Autodesk Inventor part; units mm, degrees
(part 3 of 4)
  line L1517 (59.25, 16.75) -> (45.25, 30.75) construction
  line L1518 (78.25, 16.75) -> (78.25, 30.75)
  line L1519 (64.25, 30.75) -> (64.25, 16.75)
  line L1520 (78.25, 30.75) -> (64.25, 30.75)
  line L1521 (64.25, 16.75) -> (78.25, 16.75)
  line L1522 (64.25, 16.75) -> (78.25, 30.75) construction
  line L1523 (78.25, 16.75) -> (64.25, 30.75) construction
  line L1524 (97.25, 16.75) -> (97.25, 30.75)
  line L1525 (83.25, 30.75) -> (83.25, 16.75)
  line L1526 (97.25, 30.75) -> (83.25, 30.75)
  line L1527 (83.25, 16.75) -> (97.25, 16.75)
  line L1528 (83.25, 16.75) -> (97.25, 30.75) construction
  line L1529 (97.25, 16.75) -> (83.25, 30.75) construction
  line L1530 (116.25, 16.75) -> (116.25, 30.75)
  line L1531 (102.25, 30.75) -> (102.25, 16.75)
  line L1532 (116.25, 30.75) -> (102.25, 30.75)
  line L1533 (102.25, 16.75) -> (116.25, 16.75)
  line L1534 (102.25, 16.75) -> (116.25, 30.75) construction
  line L1535 (116.25, 16.75) -> (102.25, 30.75) construction
  line L1536 (135.25, 16.75) -> (135.25, 30.75)
  line L1537 (121.25, 30.75) -> (121.25, 16.75)
  line L1538 (135.25, 30.75) -> (121.25, 30.75)
  line L1539 (121.25, 16.75) -> (135.25, 16.75)
  line L1540 (121.25, 16.75) -> (135.25, 30.75) construction
  line L1541 (135.25, 16.75) -> (121.25, 30.75) construction
  line L1542 (154.25, 16.75) -> (154.25, 30.75)
  line L1543 (140.25, 30.75) -> (140.25, 16.75)
  line L1544 (154.25, 30.75) -> (140.25, 30.75)
  line L1545 (140.25, 16.75) -> (154.25, 16.75)
  line L1546 (140.25, 16.75) -> (154.25, 30.75) construction
  line L1547 (154.25, 16.75) -> (140.25, 30.75) construction
  line L1548 (173.25, 16.75) -> (173.25, 30.75)
  line L1549 (159.25, 30.75) -> (159.25, 16.75)
  line L1550 (173.25, 30.75) -> (159.25, 30.75)
  line L1551 (159.25, 16.75) -> (173.25, 16.75)
  line L1552 (159.25, 16.75) -> (173.25, 30.75) construction
  line L1553 (173.25, 16.75) -> (159.25, 30.75) construction
  line L1554 (-64, -2.25) -> (-50, -2.25)
  line L1555 (-50, -2.25) -> (-50, 11.75)
  line L1556 (-50, 11.75) -> (-64, 11.75)
  line L1557 (-64, 11.75) -> (-64, -2.25)
  line L1558 (-64, -2.25) -> (-50, 11.75) construction
  line L1559 (-50, -2.25) -> (-64, 11.75) construction
  line L1560 (-61.625, -21.25) -> (-47.625, -21.25)
  line L1561 (-47.625, -21.25) -> (-47.625, -7.25)
  line L1562 (-47.625, -7.25) -> (-61.625, -7.25)
  line L1563 (-61.625, -7.25) -> (-61.625, -21.25)
  line L1564 (-61.625, -21.25) -> (-47.625, -7.25) construction
  line L1565 (-47.625, -21.25) -> (-61.625, -7.25) construction
  line L1566 (-56.875, -40.25) -> (-42.875, -40.25)
  line L1567 (-42.875, -40.25) -> (-42.875, -26.25)
  line L1568 (-42.875, -26.25) -> (-56.875, -26.25)
  line L1569 (-56.875, -26.25) -> (-56.875, -40.25)
  line L1570 (-56.875, -40.25) -> (-42.875, -26.25) construction
  line L1571 (-42.875, -40.25) -> (-56.875, -26.25) construction
  line L1572 (-66.375, -59.25) -> (-52.375, -59.25)
  line L1573 (-52.375, -59.25) -> (-52.375, -45.25)
  line L1574 (-52.375, -45.25) -> (-66.375, -45.25)
  line L1575 (-66.375, -45.25) -> (-66.375, -59.25)
  line L1576 (-66.375, -59.25) -> (-52.375, -45.25) construction
  line L1577 (-52.375, -59.25) -> (-66.375, -45.25) construction
  line L1578 (-42.625, -59.25) -> (-28.625, -59.25)
  line L1579 (-28.625, -59.25) -> (-28.625, -45.25)
  line L1580 (-28.625, -45.25) -> (-42.625, -45.25)
  line L1581 (-42.625, -45.25) -> (-42.625, -59.25)
  line L1582 (-42.625, -59.25) -> (-28.625, -45.25) construction
  line L1583 (-28.625, -59.25) -> (-42.625, -45.25) construction
  line L1584 (-18.875, -59.25) -> (-4.875, -59.25)
  line L1585 (-4.875, -59.25) -> (-4.875, -45.25)
  line L1586 (-4.875, -45.25) -> (-18.875, -45.25)
  line L1587 (-18.875, -45.25) -> (-18.875, -59.25)
  line L1588 (-18.875, -59.25) -> (-4.875, -45.25) construction
  line L1589 (-4.875, -59.25) -> (-18.875, -45.25) construction
  line L1590 (64.25, -59.25) -> (78.25, -59.25)
  line L1591 (78.25, -59.25) -> (78.25, -45.25)
  line L1592 (78.25, -45.25) -> (64.25, -45.25)
  line L1593 (64.25, -45.25) -> (64.25, -59.25)
  line L1594 (64.25, -59.25) -> (78.25, -45.25) construction
  line L1595 (78.25, -59.25) -> (64.25, -45.25) construction
  line L1596 (147.375, -59.25) -> (161.375, -59.25)
  line L1597 (161.375, -59.25) -> (161.375, -45.25)
  line L1598 (161.375, -45.25) -> (147.375, -45.25)
  line L1599 (147.375, -45.25) -> (147.375, -59.25)
  line L1600 (147.375, -59.25) -> (161.375, -45.25) construction
  line L1601 (161.375, -59.25) -> (147.375, -45.25) construction
  line L1602 (171.125, -59.25) -> (185.125, -59.25)
  line L1603 (185.125, -59.25) -> (185.125, -45.25)
  line L1604 (185.125, -45.25) -> (171.125, -45.25)
  line L1605 (171.125, -45.25) -> (171.125, -59.25)
  line L1606 (171.125, -59.25) -> (185.125, -45.25) construction
  line L1607 (185.125, -59.25) -> (171.125, -45.25) construction
  line L1608 (194.875, -59.25) -> (208.875, -59.25)
  line L1609 (208.875, -59.25) -> (208.875, -45.25)
  line L1610 (208.875, -45.25) -> (194.875, -45.25)
  line L1611 (194.875, -45.25) -> (194.875, -59.25)
  line L1612 (194.875, -59.25) -> (208.875, -45.25) construction
  line L1613 (208.875, -59.25) -> (194.875, -45.25) construction
  line L1614 (180.625, -40.25) -> (194.625, -40.25)
  line L1615 (194.625, -40.25) -> (194.625, -26.25)
  line L1616 (194.625, -26.25) -> (180.625, -26.25)
  line L1617 (180.625, -26.25) -> (180.625, -40.25)
  line L1618 (180.625, -40.25) -> (194.625, -26.25) construction
  line L1619 (194.625, -40.25) -> (180.625, -26.25) construction
  line L1620 (185.375, -21.25) -> (199.375, -21.25)
  line L1621 (199.375, -21.25) -> (199.375, -7.25)
  line L1622 (199.375, -7.25) -> (185.375, -7.25)
  line L1623 (185.375, -7.25) -> (185.375, -21.25)
  line L1624 (185.375, -21.25) -> (199.375, -7.25) construction
  line L1625 (199.375, -21.25) -> (185.375, -7.25) construction
  line L1626 (192.5, -2.25) -> (206.5, -2.25)
  line L1627 (206.5, -2.25) -> (206.5, 11.75)
  line L1628 (206.5, 11.75) -> (192.5, 11.75)
  line L1629 (192.5, 11.75) -> (192.5, -2.25)
  line L1630 (192.5, -2.25) -> (206.5, 11.75) construction
  line L1631 (206.5, -2.25) -> (192.5, 11.75) construction
  line L1632 (187.75, 16.75) -> (201.75, 16.75)
  line L1633 (201.75, 16.75) -> (201.75, 30.75)
  line L1634 (201.75, 30.75) -> (187.75, 30.75)
  line L1635 (187.75, 30.75) -> (187.75, 16.75)
  line L1636 (187.75, 16.75) -> (201.75, 30.75) construction
  line L1637 (201.75, 16.75) -> (187.75, 30.75) construction
  line L1638 (-40.25, -2.25) -> (-26.25, -2.25)
  line L1639 (-26.25, -2.25) -> (-26.25, 11.75)
  line L1640 (-26.25, 11.75) -> (-40.25, 11.75)
  line L1641 (-40.25, 11.75) -> (-40.25, -2.25)
  line L1642 (-40.25, -2.25) -> (-26.25, 11.75) construction
  line L1643 (-26.25, -2.25) -> (-40.25, 11.75) construction
  line L1644 (-35.5, -21.25) -> (-21.5, -21.25)
  line L1645 (-21.5, -21.25) -> (-21.5, -7.25)
  line L1646 (-21.5, -7.25) -> (-35.5, -7.25)
  line L1647 (-35.5, -7.25) -> (-35.5, -21.25)
  line L1648 (-35.5, -21.25) -> (-21.5, -7.25) construction
  line L1649 (-21.5, -21.25) -> (-35.5, -7.25) construction
  line L1650 (-26, -40.25) -> (-12, -40.25)
  line L1651 (-12, -40.25) -> (-12, -26.25)
  line L1652 (-12, -26.25) -> (-26, -26.25)
  line L1653 (-26, -26.25) -> (-26, -40.25)
  line L1654 (-26, -40.25) -> (-12, -26.25) construction
  line L1655 (-12, -40.25) -> (-26, -26.25) construction
  line L1656 (-21.25, -2.25) -> (-7.25, -2.25)
  line L1657 (-21.25, 11.75) -> (-21.25, -2.25)
  line L1658 (-7.25, -2.25) -> (-7.25, 11.75)
  line L1659 (-7.25, 11.75) -> (-21.25, 11.75)
  line L1660 (-21.25, -2.25) -> (-7.25, 11.75) construction
  line L1661 (-7.25, -2.25) -> (-21.25, 11.75) construction
  line L1662 (-2.25, -2.25) -> (11.75, -2.25)
  line L1663 (-2.25, 11.75) -> (-2.25, -2.25)
  line L1664 (11.75, -2.25) -> (11.75, 11.75)
  line L1665 (11.75, 11.75) -> (-2.25, 11.75)
  line L1666 (-2.25, -2.25) -> (11.75, 11.75) construction
  line L1667 (11.75, -2.25) -> (-2.25, 11.75) construction
  line L1668 (16.75, -2.25) -> (30.75, -2.25)
  line L1669 (16.75, 11.75) -> (16.75, -2.25)
  line L1670 (30.75, -2.25) -> (30.75, 11.75)
  line L1671 (30.75, 11.75) -> (16.75, 11.75)
  line L1672 (16.75, -2.25) -> (30.75, 11.75) construction
  line L1673 (30.75, -2.25) -> (16.75, 11.75) construction
  line L1674 (35.75, -2.25) -> (49.75, -2.25)
  line L1675 (35.75, 11.75) -> (35.75, -2.25)
  line L1676 (49.75, -2.25) -> (49.75, 11.75)
  line L1677 (49.75, 11.75) -> (35.75, 11.75)
  line L1678 (35.75, -2.25) -> (49.75, 11.75) construction
  line L1679 (49.75, -2.25) -> (35.75, 11.75) construction
  line L1680 (54.75, -2.25) -> (68.75, -2.25)
  line L1681 (54.75, 11.75) -> (54.75, -2.25)
  line L1682 (68.75, -2.25) -> (68.75, 11.75)
  line L1683 (68.75, 11.75) -> (54.75, 11.75)
  line L1684 (54.75, -2.25) -> (68.75, 11.75) construction
  line L1685 (68.75, -2.25) -> (54.75, 11.75) construction
  line L1686 (73.75, -2.25) -> (87.75, -2.25)
  line L1687 (73.75, 11.75) -> (73.75, -2.25)
  line L1688 (87.75, -2.25) -> (87.75, 11.75)
  line L1689 (87.75, 11.75) -> (73.75, 11.75)
  line L1690 (73.75, -2.25) -> (87.75, 11.75) construction
  line L1691 (87.75, -2.25) -> (73.75, 11.75) construction
  line L1692 (92.75, -2.25) -> (106.75, -2.25)
  line L1693 (92.75, 11.75) -> (92.75, -2.25)
  line L1694 (106.75, -2.25) -> (106.75, 11.75)
  line L1695 (106.75, 11.75) -> (92.75, 11.75)
  line L1696 (92.75, -2.25) -> (106.75, 11.75) construction
  line L1697 (106.75, -2.25) -> (92.75, 11.75) construction
  line L1698 (111.75, -2.25) -> (125.75, -2.25)
  line L1699 (111.75, 11.75) -> (111.75, -2.25)
  line L1700 (125.75, -2.25) -> (125.75, 11.75)
  line L1701 (125.75, 11.75) -> (111.75, 11.75)
  line L1702 (111.75, -2.25) -> (125.75, 11.75) construction
  line L1703 (125.75, -2.25) -> (111.75, 11.75) construction
  line L1704 (130.75, -2.25) -> (144.75, -2.25)
  line L1705 (130.75, 11.75) -> (130.75, -2.25)
  line L1706 (144.75, -2.25) -> (144.75, 11.75)
  line L1707 (144.75, 11.75) -> (130.75, 11.75)
  line L1708 (130.75, -2.25) -> (144.75, 11.75) construction
  line L1709 (144.75, -2.25) -> (130.75, 11.75) construction
  line L1710 (149.75, -2.25) -> (163.75, -2.25)
  line L1711 (149.75, 11.75) -> (149.75, -2.25)
  line L1712 (163.75, -2.25) -> (163.75, 11.75)
  line L1713 (163.75, 11.75) -> (149.75, 11.75)
  line L1714 (149.75, -2.25) -> (163.75, 11.75) construction
  line L1715 (163.75, -2.25) -> (149.75, 11.75) construction
  line L1716 (168.75, -2.25) -> (182.75, -2.25)
  line L1717 (168.75, 11.75) -> (168.75, -2.25)
  line L1718 (182.75, -2.25) -> (182.75, 11.75)
  line L1719 (182.75, 11.75) -> (168.75, 11.75)
  line L1720 (168.75, -2.25) -> (182.75, 11.75) construction
  line L1721 (182.75, -2.25) -> (168.75, 11.75) construction
  line L1722 (-16.5, -21.25) -> (-2.5, -21.25)
  line L1723 (-16.5, -7.25) -> (-16.5, -21.25)
  line L1724 (-2.5, -7.25) -> (-16.5, -7.25)
  line L1725 (-2.5, -21.25) -> (-2.5, -7.25)
  line L1726 (-16.5, -21.25) -> (-2.5, -7.25) construction
  line L1727 (-2.5, -21.25) -> (-16.5, -7.25) construction
  line L1728 (2.5, -21.25) -> (16.5, -21.25)
  line L1729 (2.5, -7.25) -> (2.5, -21.25)
  line L1730 (16.5, -7.25) -> (2.5, -7.25)
  line L1731 (16.5, -21.25) -> (16.5, -7.25)
  line L1732 (2.5, -21.25) -> (16.5, -7.25) construction
  line L1733 (16.5, -21.25) -> (2.5, -7.25) construction
  line L1734 (21.5, -21.25) -> (35.5, -21.25)
  line L1735 (21.5, -7.25) -> (21.5, -21.25)
  line L1736 (35.5, -7.25) -> (21.5, -7.25)
  line L1737 (35.5, -21.25) -> (35.5, -7.25)
  line L1738 (21.5, -21.25) -> (35.5, -7.25) construction
  line L1739 (35.5, -21.25) -> (21.5, -7.25) construction
  line L1740 (40.5, -21.25) -> (54.5, -21.25)
  line L1741 (40.5, -7.25) -> (40.5, -21.25)
  line L1742 (54.5, -7.25) -> (40.5, -7.25)
  line L1743 (54.5, -21.25) -> (54.5, -7.25)
  line L1744 (40.5, -21.25) -> (54.5, -7.25) construction
  line L1745 (54.5, -21.25) -> (40.5, -7.25) construction
  line L1746 (59.5, -21.25) -> (73.5, -21.25)
  line L1747 (59.5, -7.25) -> (59.5, -21.25)
  line L1748 (73.5, -7.25) -> (59.5, -7.25)
  line L1749 (73.5, -21.25) -> (73.5, -7.25)
  line L1750 (59.5, -21.25) -> (73.5, -7.25) construction
  line L1751 (73.5, -21.25) -> (59.5, -7.25) construction
  line L1752 (78.5, -21.25) -> (92.5, -21.25)
  line L1753 (78.5, -7.25) -> (78.5, -21.25)
  line L1754 (92.5, -7.25) -> (78.5, -7.25)
  line L1755 (92.5, -21.25) -> (92.5, -7.25)
  line L1756 (78.5, -21.25) -> (92.5, -7.25) construction
  line L1757 (92.5, -21.25) -> (78.5, -7.25) construction
  line L1758 (97.5, -21.25) -> (111.5, -21.25)
  line L1759 (97.5, -7.25) -> (97.5, -21.25)
  line L1760 (111.5, -7.25) -> (97.5, -7.25)
  line L1761 (111.5, -21.25) -> (111.5, -7.25)
  line L1762 (97.5, -21.25) -> (111.5, -7.25) construction
  line L1763 (111.5, -21.25) -> (97.5, -7.25) construction
  line L1764 (116.5, -21.25) -> (130.5, -21.25)
  line L1765 (116.5, -7.25) -> (116.5, -21.25)
  line L1766 (130.5, -7.25) -> (116.5, -7.25)
  line L1767 (130.5, -21.25) -> (130.5, -7.25)
  line L1768 (116.5, -21.25) -> (130.5, -7.25) construction
  line L1769 (130.5, -21.25) -> (116.5, -7.25) construction
  line L1770 (135.5, -21.25) -> (149.5, -21.25)
  line L1771 (135.5, -7.25) -> (135.5, -21.25)
  line L1772 (149.5, -7.25) -> (135.5, -7.25)
  line L1773 (149.5, -21.25) -> (149.5, -7.25)
  line L1774 (135.5, -21.25) -> (149.5, -7.25) construction
  line L1775 (149.5, -21.25) -> (135.5, -7.25) construction
  line L1776 (154.5, -21.25) -> (168.5, -21.25)
  line L1777 (154.5, -7.25) -> (154.5, -21.25)
  line L1778 (168.5, -7.25) -> (154.5, -7.25)
  line L1779 (168.5, -21.25) -> (168.5, -7.25)
  line L1780 (154.5, -21.25) -> (168.5, -7.25) construction
  line L1781 (168.5, -21.25) -> (154.5, -7.25) construction
  line L1782 (-7, -40.25) -> (7, -40.25)
  line L1783 (-7, -26.25) -> (-7, -40.25)
  line L1784 (7, -26.25) -> (-7, -26.25)
  line L1785 (7, -40.25) -> (7, -26.25)
  line L1786 (-7, -40.25) -> (7, -26.25) construction
  line L1787 (7, -40.25) -> (-7, -26.25) construction
  line L1788 (12, -40.25) -> (26, -40.25)
  line L1789 (12, -26.25) -> (12, -40.25)
  line L1790 (26, -26.25) -> (12, -26.25)
  line L1791 (26, -40.25) -> (26, -26.25)
  line L1792 (12, -40.25) -> (26, -26.25) construction
  line L1793 (26, -40.25) -> (12, -26.25) construction
  line L1794 (31, -40.25) -> (45, -40.25)
  line L1795 (31, -26.25) -> (31, -40.25)
  line L1796 (45, -26.25) -> (31, -26.25)
  line L1797 (45, -40.25) -> (45, -26.25)
  line L1798 (31, -40.25) -> (45, -26.25) construction
  line L1799 (45, -40.25) -> (31, -26.25) construction
  line L1800 (50, -40.25) -> (64, -40.25)
  line L1801 (50, -26.25) -> (50, -40.25)
  line L1802 (64, -26.25) -> (50, -26.25)
  line L1803 (64, -40.25) -> (64, -26.25)
  line L1804 (50, -40.25) -> (64, -26.25) construction
  line L1805 (64, -40.25) -> (50, -26.25) construction
  line L1806 (69, -40.25) -> (83, -40.25)
  line L1807 (69, -26.25) -> (69, -40.25)
  line L1808 (83, -26.25) -> (69, -26.25)
  line L1809 (83, -40.25) -> (83, -26.25)
  line L1810 (69, -40.25) -> (83, -26.25) construction
  line L1811 (83, -40.25) -> (69, -26.25) construction
  line L1812 (88, -40.25) -> (102, -40.25)
  line L1813 (88, -26.25) -> (88, -40.25)
  line L1814 (102, -26.25) -> (88, -26.25)
  line L1815 (102, -40.25) -> (102, -26.25)
  line L1816 (88, -40.25) -> (102, -26.25) construction
  line L1817 (102, -40.25) -> (88, -26.25) construction
  line L1818 (107, -40.25) -> (121, -40.25)
  line L1819 (107, -26.25) -> (107, -40.25)
  line L1820 (121, -26.25) -> (107, -26.25)
  line L1821 (121, -40.25) -> (121, -26.25)
  line L1822 (107, -40.25) -> (121, -26.25) construction
  line L1823 (121, -40.25) -> (107, -26.25) construction
  line L1824 (126, -40.25) -> (140, -40.25)
  line L1825 (126, -26.25) -> (126, -40.25)
  line L1826 (140, -26.25) -> (126, -26.25)
  line L1827 (140, -40.25) -> (140, -26.25)
  line L1828 (126, -40.25) -> (140, -26.25) construction
  line L1829 (140, -40.25) -> (126, -26.25) construction
  line L1830 (145, -40.25) -> (159, -40.25)
  line L1831 (145, -26.25) -> (145, -40.25)
  line L1832 (159, -26.25) -> (145, -26.25)
  line L1833 (159, -40.25) -> (159, -26.25)
  line L1834 (145, -40.25) -> (159, -26.25) construction
  line L1835 (159, -40.25) -> (145, -26.25) construction
  point P0 (107.46, 92.5006)
  point P1 (-61.75, 52.25)
  point P2 (-23.75, 52.25)
  point P3 (-4.75, 52.25)
  point P4 (14.25, 52.25)
  point P5 (33.25, 52.25)
  point P6 (61.75, 52.25)
  point P7 (147.25, 52.25)
  point P8 (-204.25, 23.75)
  point P9 (-147.25, 23.75)
  point P10 (-147.25, -4.75)
  point P11 (-147.25, -42.75)
  point P12 (-123.5, -52.25)
  point P13 (-104.5, -52.25)
  point P14 (-85.5, -52.25)
  point P15 (-104.5, -33.25)
  point P16 (-123.5, 23.75)
  point P17 (-61.75, 23.75)
  point P18 (-57, 4.75)
  point P19 (-54.625, -14.25)
  point P20 (-49.875, -33.25)
  point P21 (-59.375, -52.25)
  point P22 (-35.625, -52.25)
  point P23 (-11.875, -52.25)
  point P24 (71.25, -52.25)
  point P25 (154.375, -52.25)
  point P26 (178.125, -52.25)
  point P27 (201.875, -52.25)
  point P28 (187.625, -33.25)
  point P29 (192.375, -14.25)
  point P30 (199.5, 4.75)
  point P31 (194.75, 23.75)
  point P32 (-33.25, 4.75)
  point P33 (-28.5, -14.25)
  point P34 (-19, -33.25)
  dimension "d0" = 0.7
  dimension "d1" = 0.7
  dimension "d2" = 14
  dimension "d3" = 14
  dimension "d4" = 14
  dimension "d5" = 14
  dimension "d6" = 14
  dimension "d7" = 14
  dimension "d8" = 14
  dimension "d9" = 14
  dimension "d10" = 14
  dimension "d11" = 14
  dimension "d12" = 14
  dimension "d13" = 14
  dimension "d16" = 19
  dimension "d21" = 14
  dimension "d22" = 14
  dimension "d25" = 19
  dimension "d30" = 14
  dimension "d31" = 14
  dimension "d34" = 19
  dimension "d37" = 19
  dimension "d40" = 14
  dimension "d41" = 14
  dimension "d42" = 14
  dimension "d43" = 14
  dimension "d44" = 14
  dimension "d45" = 14
  dimension "d46" = 14
  dimension "d47" = 14
  dimension "d48" = 14
  dimension "d49" = 14
  dimension "d50" = 14
  dimension "d51" = 14
  dimension "d52" = 14
  dimension "d53" = 14
  dimension "d54" = 14
  dimension "d55" = 14
  dimension "d58" = 19
  dimension "d61" = 19
  dimension "d64" = 14
  dimension "d65" = 14
  dimension "d68" = 19
  dimension "d73" = 14
  dimension "d74" = 14
  dimension "d75" = 14
  dimension "d76" = 14
  dimension "d77" = 14
  dimension "d78" = 14
  dimension "d79" = 14
  dimension "d80" = 14
  dimension "d81" = 14
  dimension "d82" = 14
  dimension "d83" = 14
  dimension "d84" = 14
  dimension "d85" = 14
  dimension "d86" = 14
  dimension "d87" = 14
  dimension "d88" = 14
  dimension "d89" = 14
  dimension "d90" = 14
  dimension "d91" = 14
  dimension "d92" = 14
  dimension "d93" = 14
  constraints: 1226 end point, 68 midpoint, 68 parallel, 43 horizontal, 38 perpendicular, 10 collinear, 5 point on line, 3 vertical, 660 other
  measures "d0" distance of L4.start L12.end
  measures "d1" distance of L4.end L15.end
  measures "d2" distance of L1232.end L1231.end
  measures "d3" distance of L1231.end L1230.end
  measures "d4" distance of L1238.end L1237.end
  measures "d5" distance of L1237.end L1236.end
  measures "d6" distance of L1244.end L1243.end
  measures "d7" distance of L1243.end L1242.end
  measures "d8" distance of L1250.end L1249.end
  measures "d9" distance of L1249.end L1248.end
  measures "d10" distance of L1256.end L1255.end
  measures "d11" distance of L1255.end L1254.end
  measures "d12" distance of L1262.end L1261.end
  measures "d13" distance of L1261.end L1260.end
  measures "d16" distance of L1260.start L1266.start
  measures "d21" distance of L1286.end L1285.end
  measures "d22" distance of L1285.end L1284.end
  measures "d25" distance of L1284.end L1290.start
  measures "d30" distance of L1310.end L1309.end
  measures "d31" distance of L1309.end L1308.end
  measures "d34" distance of L1309.end L1314.start
  measures "d37" distance of L1309.end L1326.start
  measures "d40" distance of L1400.end L1399.end
  measures "d41" distance of L1399.end L1398.end
  measures "d42" distance of L1406.end L1405.end
  measures "d43" distance of L1405.end L1404.end
  measures "d44" distance of L1412.end L1411.end
  measures "d45" distance of L1411.end L1410.end
  measures "d46" distance of L1418.end L1417.end
  measures "d47" distance of L1417.end L1416.end
  measures "d48" distance of L1424.end L1423.end
  measures "d49" distance of L1423.end L1422.end
  measures "d50" distance of L1430.end L1429.end
  measures "d51" distance of L1429.end L1428.end
  measures "d52" distance of L1435.end L1436.end
  measures "d53" distance of L1434.end L1435.end
  measures "d54" distance of L1442.end L1441.end
  measures "d55" distance of L1441.end L1440.end
  measures "d58" distance of L1442.end L1446.end
  measures "d61" distance of L1442.end L1458.end
  measures "d64" distance of L1478.end L1477.end
  measures "d65" distance of L1477.end L1476.end
  measures "d68" distance of L1476.end L1482.start
  measures "d73" distance of L1556.end L1555.end
  measures "d74" distance of L1555.end L1554.end
  measures "d75" distance of L1562.end L1561.end
  measures "d76" distance of L1561.end L1560.end
  measures "d77" distance of L1568.end L1567.end
  measures "d78" distance of L1567.end L1566.end
  measures "d79" distance of L1574.end L1573.end
  measures "d80" distance of L1573.end L1572.end
  measures "d81" distance of L1580.end L1579.end
  measures "d82" distance of L1579.end L1578.end
  measures "d83" distance of L1586.end L1585.end
  measures "d84" distance of L1585.end L1584.end
  measures "d85" distance of L1592.end L1591.end
  measures "d86" distance of L1591.end L1590.end
  measures "d87" distance of L1598.end L1597.end
  measures "d88" distance of L1597.end L1596.end
  measures "d89" distance of L1604.end L1603.end
  measures "d90" distance of L1603.end L1602.end
  measures "d91" distance of L1610.end L1609.end
  measures "d92" distance of L1609.end L1608.end
  measures "d93" distance of L1616.end L1615.end
extrude "Extrusion1" add sketch "Sketch1" against normal blind 1.5 contours A3 L3 A2 L2 A1 L1 A0 L0 | A4 | A5 | A6 | A7 | A8 | A9 | A10 | A11 | A12 | A13 | A14 | A15 | A16 | A17 | A18 | A19 | A20 | A21 | A22 | A23 | A24 | A25 | A26 | A27
sketch "Sketch2" plane through (-107.46, -92.5006, 10.9251) normal (0, 0, 1) x (1, 0, 0)
  arc A0 (-216.125, 61.75) -> (-220.875, 57) centre (-216.125, 57) ccw construction
  line L0 (-216.125, -61.75) -> (216.125, -61.75) construction
  line L1 (-220.875, 57) -> (-220.875, -57) construction
  arc A1 (220.875, 57) -> (216.125, 61.75) centre (216.125, 57) ccw construction
  line L2 (216.125, 61.75) -> (-216.125, 61.75) construction
  line L3 (-213.77, 61.75) -> (-213.77, -61.75) construction
  line L4 (-211.25, 30.75) -> (-197.25, 30.75) construction
  line L5 (-213.77, 35.75) -> (-212.3378, 39.685)
  line L6 (-205.2313, 59.21) -> (-202.7313, 59.21)
  line L7 (-213.77, 35.75) -> (-211.27, 35.75)
  line L8 (-210.231, 59.21) -> (-185.2654, 59.21) construction
  line L9 (-133.77, 35.75) -> (-108.8044, 35.75) construction
  line L10 (-128.77, 35.75) -> (-133.77, 35.75)
  line L11 (-123.77, 35.75) -> (-98.8044, 35.75) construction
  line L12 (-123.77, 35.75) -> (-118.77, 35.75)
  line L13 (-113.77, 35.75) -> (-88.8044, 35.75) construction
  line L14 (-108.77, 35.75) -> (-113.77, 35.75)
  line L15 (-103.77, 35.75) -> (-78.8044, 35.75) construction
  line L16 (-98.77, 35.75) -> (-103.77, 35.75)
  line L17 (-88.77, 35.75) -> (-93.77, 35.75)
  line L18 (-78.77, 35.75) -> (-83.77, 35.75)
  line L19 (-77.34, 41.535) -> (-77.34, 39.685) construction
  line L20 (-212.3378, 39.685) -> (-209.8378, 39.685)
  line L21 (-211.6644, 41.535) -> (-209.1644, 41.535)
  line L22 (-132.3378, 39.685) -> (-77.34, 39.685)
  line L23 (-77.34, 39.685) -> (-78.7722, 35.75)
  line L24 (-128.77, 35.75) -> (-123.77, 35.75)
  line L25 (-118.77, 35.75) -> (-113.77, 35.75)
  line L26 (-108.77, 35.75) -> (-103.77, 35.75)
  line L27 (-98.77, 35.75) -> (-93.77, 35.75)
  line L28 (-88.77, 35.75) -> (-83.77, 35.75)
  line L29 (-132.3378, 39.685) -> (-133.77, 35.75)
  line L30 (-211.6644, 41.535) -> (-205.2313, 59.21)
  line L31 (-129.54, 41.535) -> (-129.54, 59.315) construction
  line L32 (-129.54, 59.0513) -> (-131.39, 59.0513) construction
  line L33 (-129.54, 59.0513) -> (-127.69, 59.0513) construction
  line L34 (-131.39, 61.75) -> (-131.39, 56.0264) construction
  line L35 (-130.2313, 59.21) -> (220.875, 59.21) construction
  line L36 (-131.39, 56.0264) -> (-131.39, 39.685) construction
  line L37 (-211.27, 35.75) -> (-209.8378, 39.685) construction
  line L38 (-209.1644, 41.535) -> (-202.7313, 59.21) construction
  line L39 (-211.27, 35.75) -> (-209.8378, 39.685)
  line L40 (-209.1644, 41.535) -> (-202.7313, 59.21)
  line L41 (-213.77, 59.21) -> (-131.39, 59.21) construction
  line L42 (-200.2313, 59.21) -> (-197.7313, 59.21)
  line L43 (-204.1644, 41.535) -> (-197.7313, 59.21) construction
  line L44 (-204.1644, 41.535) -> (-197.7313, 59.21)
  line L45 (-206.6644, 41.535) -> (-200.2313, 59.21)
  line L46 (-206.6644, 41.535) -> (-204.1644, 41.535)
  line L47 (-207.3378, 39.685) -> (-204.8378, 39.685)
  line L48 (-206.27, 35.75) -> (-204.8378, 39.685) construction
  line L49 (-206.27, 35.75) -> (-204.8378, 39.685)
  line L50 (-208.77, 35.75) -> (-207.3378, 39.685)
  line L51 (-208.77, 35.75) -> (-206.27, 35.75)
  line L52 (-195.2313, 59.21) -> (-192.7313, 59.21)
  line L53 (-199.1644, 41.535) -> (-192.7313, 59.21) construction
  line L54 (-199.1644, 41.535) -> (-192.7313, 59.21)
  line L55 (-201.6644, 41.535) -> (-195.2313, 59.21)
  line L56 (-201.6644, 41.535) -> (-199.1644, 41.535)
  line L57 (-202.3378, 39.685) -> (-199.8378, 39.685)
  line L58 (-201.27, 35.75) -> (-199.8378, 39.685) construction
  line L59 (-201.27, 35.75) -> (-199.8378, 39.685)
  line L60 (-203.77, 35.75) -> (-202.3378, 39.685)
  line L61 (-203.77, 35.75) -> (-201.27, 35.75)
  line L62 (-190.2313, 59.21) -> (-187.7313, 59.21)
  line L63 (-194.1644, 41.535) -> (-187.7313, 59.21) construction
  line L64 (-194.1644, 41.535) -> (-187.7313, 59.21)
  line L65 (-196.6644, 41.535) -> (-190.2313, 59.21)
  line L66 (-196.6644, 41.535) -> (-194.1644, 41.535)
  line L67 (-197.3378, 39.685) -> (-194.8378, 39.685)
  line L68 (-196.27, 35.75) -> (-194.8378, 39.685) construction
  line L69 (-196.27, 35.75) -> (-194.8378, 39.685)
  line L70 (-198.77, 35.75) -> (-197.3378, 39.685)
  line L71 (-198.77, 35.75) -> (-196.27, 35.75)
  line L72 (-185.2313, 59.21) -> (-182.7313, 59.21)
  line L73 (-189.1644, 41.535) -> (-182.7313, 59.21) construction
  line L74 (-189.1644, 41.535) -> (-182.7313, 59.21)
  line L75 (-191.6644, 41.535) -> (-185.2313, 59.21)
  line L76 (-191.6644, 41.535) -> (-189.1644, 41.535)
  line L77 (-192.3378, 39.685) -> (-189.8378, 39.685)
  line L78 (-191.27, 35.75) -> (-189.8378, 39.685) construction
  line L79 (-191.27, 35.75) -> (-189.8378, 39.685)
  line L80 (-193.77, 35.75) -> (-192.3378, 39.685)
  line L81 (-193.77, 35.75) -> (-191.27, 35.75)
  line L82 (-180.2313, 59.21) -> (-177.7313, 59.21)
  line L83 (-184.1644, 41.535) -> (-177.7313, 59.21) construction
  line L84 (-184.1644, 41.535) -> (-177.7313, 59.21)
  line L85 (-186.6644, 41.535) -> (-180.2313, 59.21)
  line L86 (-186.6644, 41.535) -> (-184.1644, 41.535)
  line L87 (-187.3378, 39.685) -> (-184.8378, 39.685)
  line L88 (-186.27, 35.75) -> (-184.8378, 39.685) construction
  line L89 (-186.27, 35.75) -> (-184.8378, 39.685)
  line L90 (-188.77, 35.75) -> (-187.3378, 39.685)
  line L91 (-188.77, 35.75) -> (-186.27, 35.75)
  line L92 (-175.2313, 59.21) -> (-172.7313, 59.21)
  line L93 (-179.1644, 41.535) -> (-172.7313, 59.21) construction
  line L94 (-179.1644, 41.535) -> (-172.7313, 59.21)
  line L95 (-181.6644, 41.535) -> (-175.2313, 59.21)
  line L96 (-181.6644, 41.535) -> (-179.1644, 41.535)
  line L97 (-182.3378, 39.685) -> (-179.8378, 39.685)
  line L98 (-181.27, 35.75) -> (-179.8378, 39.685) construction
  line L99 (-181.27, 35.75) -> (-179.8378, 39.685)
  line L100 (-183.77, 35.75) -> (-182.3378, 39.685)
  line L101 (-183.77, 35.75) -> (-181.27, 35.75)
  line L102 (-170.2313, 59.21) -> (-167.7313, 59.21)
  line L103 (-174.1644, 41.535) -> (-167.7313, 59.21) construction
  line L104 (-174.1644, 41.535) -> (-167.7313, 59.21)
  line L105 (-176.6644, 41.535) -> (-170.2313, 59.21)
  line L106 (-176.6644, 41.535) -> (-174.1644, 41.535)
  line L107 (-177.3378, 39.685) -> (-174.8378, 39.685)
  line L108 (-176.27, 35.75) -> (-174.8378, 39.685) construction
  line L109 (-176.27, 35.75) -> (-174.8378, 39.685)
  line L110 (-178.77, 35.75) -> (-177.3378, 39.685)
  line L111 (-178.77, 35.75) -> (-176.27, 35.75)
  line L112 (-165.2313, 59.21) -> (-162.7313, 59.21)
  line L113 (-169.1644, 41.535) -> (-162.7313, 59.21) construction
  line L114 (-169.1644, 41.535) -> (-162.7313, 59.21)
  line L115 (-171.6644, 41.535) -> (-165.2313, 59.21)
  line L116 (-171.6644, 41.535) -> (-169.1644, 41.535)
  line L117 (-172.3378, 39.685) -> (-169.8378, 39.685)
  line L118 (-171.27, 35.75) -> (-169.8378, 39.685) construction
  line L119 (-171.27, 35.75) -> (-169.8378, 39.685)
  line L120 (-173.77, 35.75) -> (-172.3378, 39.685)
  line L121 (-173.77, 35.75) -> (-171.27, 35.75)
  line L122 (-160.2313, 59.21) -> (-157.7313, 59.21)
  line L123 (-164.1644, 41.535) -> (-157.7313, 59.21) construction
  line L124 (-164.1644, 41.535) -> (-157.7313, 59.21)
  line L125 (-166.6644, 41.535) -> (-160.2313, 59.21)
  line L126 (-166.6644, 41.535) -> (-164.1644, 41.535)
  line L127 (-167.3378, 39.685) -> (-164.8378, 39.685)
  line L128 (-166.27, 35.75) -> (-164.8378, 39.685) construction
  line L129 (-166.27, 35.75) -> (-164.8378, 39.685)
  line L130 (-168.77, 35.75) -> (-167.3378, 39.685)
  line L131 (-168.77, 35.75) -> (-166.27, 35.75)
  line L132 (-155.2313, 59.21) -> (-152.7313, 59.21)
  line L133 (-159.1644, 41.535) -> (-152.7313, 59.21) construction
  line L134 (-159.1644, 41.535) -> (-152.7313, 59.21)
  line L135 (-161.6644, 41.535) -> (-155.2313, 59.21)
  line L136 (-161.6644, 41.535) -> (-159.1644, 41.535)
  line L137 (-162.3378, 39.685) -> (-159.8378, 39.685)
  line L138 (-161.27, 35.75) -> (-159.8378, 39.685) construction
  line L139 (-161.27, 35.75) -> (-159.8378, 39.685)
  line L140 (-163.77, 35.75) -> (-162.3378, 39.685)
  line L141 (-163.77, 35.75) -> (-161.27, 35.75)
  line L142 (-150.2313, 59.21) -> (-147.7313, 59.21)
  line L143 (-154.1644, 41.535) -> (-147.7313, 59.21) construction
  line L144 (-154.1644, 41.535) -> (-147.7313, 59.21)
  line L145 (-156.6644, 41.535) -> (-150.2313, 59.21)
  line L146 (-156.6644, 41.535) -> (-154.1644, 41.535)
  line L147 (-157.3378, 39.685) -> (-154.8378, 39.685)
  line L148 (-156.27, 35.75) -> (-154.8378, 39.685) construction
  line L149 (-156.27, 35.75) -> (-154.8378, 39.685)
  line L150 (-158.77, 35.75) -> (-157.3378, 39.685)
  line L151 (-158.77, 35.75) -> (-156.27, 35.75)
  line L152 (-145.2313, 59.21) -> (-142.7313, 59.21)
  line L153 (-149.1644, 41.535) -> (-142.7313, 59.21) construction
  line L154 (-149.1644, 41.535) -> (-142.7313, 59.21)
  line L155 (-151.6644, 41.535) -> (-145.2313, 59.21)
  line L156 (-151.6644, 41.535) -> (-149.1644, 41.535)
  line L157 (-152.3378, 39.685) -> (-149.8378, 39.685)
  line L158 (-151.27, 35.75) -> (-149.8378, 39.685) construction
  line L159 (-151.27, 35.75) -> (-149.8378, 39.685)
  line L160 (-153.77, 35.75) -> (-152.3378, 39.685)
  line L161 (-153.77, 35.75) -> (-151.27, 35.75)
  line L162 (-140.2313, 59.21) -> (-137.7313, 59.21)
  line L163 (-144.1644, 41.535) -> (-137.7313, 59.21) construction
  line L164 (-144.1644, 41.535) -> (-137.7313, 59.21)
  line L165 (-146.6644, 41.535) -> (-140.2313, 59.21)
  line L166 (-146.6644, 41.535) -> (-144.1644, 41.535)
  line L167 (-147.3378, 39.685) -> (-144.8378, 39.685)
  line L168 (-146.27, 35.75) -> (-144.8378, 39.685) construction
  line L169 (-146.27, 35.75) -> (-144.8378, 39.685)
  line L170 (-148.77, 35.75) -> (-147.3378, 39.685)
  line L171 (-148.77, 35.75) -> (-146.27, 35.75)
  line L172 (-135.2313, 59.21) -> (-132.7313, 59.21)
  line L173 (-139.1644, 41.535) -> (-132.7313, 59.21) construction
  line L174 (-139.1644, 41.535) -> (-132.7313, 59.21)
  line L175 (-141.6644, 41.535) -> (-135.2313, 59.21)
  line L176 (-141.6644, 41.535) -> (-139.1644, 41.535)
  line L177 (-142.3378, 39.685) -> (-139.8378, 39.685)
  line L178 (-141.27, 35.75) -> (-139.8378, 39.685) construction
  line L179 (-141.27, 35.75) -> (-139.8378, 39.685)
  line L180 (-143.77, 35.75) -> (-142.3378, 39.685)
  line L181 (-143.77, 35.75) -> (-141.27, 35.75)
  line L182 (-137.338, 39.685) -> (-138.7702, 35.75)
  line L183 (-137.338, 39.685) -> (-133.1505, 39.685) construction
  line L184 (-138.7702, 35.75) -> (-136.2702, 35.75)
  line L185 (-136.2702, 35.75) -> (-134.838, 39.685)
  line L186 (-134.838, 39.685) -> (-137.338, 39.685)
  line L187 (-136.6647, 41.535) -> (-131.39, 56.027)
  line L188 (-136.6647, 41.535) -> (-121.2426, 41.535) construction
  line L189 (-131.39, 56.027) -> (-131.39, 49.1583)
  line L190 (-136.6647, 41.535) -> (-134.1647, 41.535)
  line L191 (-134.1647, 41.535) -> (-131.39, 49.1583)
  line L192 (-207.731, 59.21) -> (-213.77, 42.618)
  line L193 (-207.731, 59.21) -> (-190.0741, 59.21) construction
  line L194 (-207.731, 59.21) -> (-210.231, 59.21)
  line L195 (-210.231, 59.21) -> (-213.77, 49.4867)
  line L196 (-213.77, 49.4867) -> (-213.77, 42.618)
  line L197 (-212.731, 59.21) -> (-209.6932, 59.21) construction
  dimension "d159" = 1.85
  dimension "d171" = 1.85
  dimension "d172" = 180
  dimension "d175" = 5
  dimension "d180" = 110
  dimension "d181" = 2.5
  dimension "d182" = 70
  dimension "d183" = 110
  dimension "d184" = 2.5
  dimension "d185" = 110
  constraints: 386 end point, 41 point on line, 8 horizontal, 5 collinear, 4 equal length, 3 perpendicular, 2 parallel, 2 point on circle, 1 centre point, 252 other
  measures "d159" distance of L19.start L19.end
  measures "d171" distance of L32.start L32.end
  measures "d172" angle of L32 L33
  measures "d175" distance of L5.start L50.start
  measures "d180" angle of L182 L183
  measures "d181" distance of L182.end L184.end
  measures "d182" angle of L188 L187
  measures "d183" angle of L192 L193
  measures "d184" distance of L192.start L8.start
  measures "d185" angle of L195 L194
extrude "Extrusion3" cut sketch "Sketch2" against normal blind 1.5